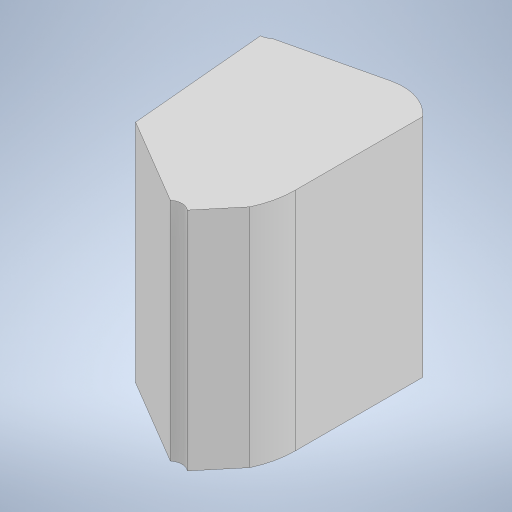
# Autodesk Inventor part: Part1
Saved by Autodesk Inventor 2024.1 (Build 281209000, 209)
## iProperties
Created: 2024-01-20
Part Number: Part1
Material: Generic
Document SubType Name: Modeling
Designer: vg3
Density: 1 g/cm^3
Appearance: Default
Author: vg3
Autodesk Inventor part; units mm, degrees
ref_plane "YZ Plane" through (0, 0, 0) normal (1, 0, 0) x (0, 1, 0)
ref_plane "XZ Plane" through (0, 0, 0) normal (0, 1, 0) x (-1, 0, 0)
ref_plane "XY Plane" through (0, 0, 0) normal (0, 0, 1) x (1, 0, 0)
sketch "Sketch1" plane through (0, 0, 0) normal (0, 1, 0) x (-1, 0, 0)
  line L0 (7.2314, 12.2227) -> (8.6145, -3.2023)
  arc A0 (8.6145, -3.2023) -> (7.6223, -3.6232) centre (8.7714, -4.952) ccw
  line L1 (7.6223, -3.6232) -> (-3.1421, -6.1489)
  arc A1 (-8.374, -4.4651) -> (-3.1421, -6.1489) centre (-4.3594, -0.9611) ccw
  line L2 (-8.374, -4.4651) -> (-8.374, 9.8774)
  arc A2 (-7.4419, 14.0569) -> (-8.374, 9.8774) centre (1.4622, 9.8774) ccw
  line L3 (-7.4419, 14.0569) -> (-4.2604, 17.8775)
  arc A3 (-4.2604, 17.8775) -> (-2.3303, 17.8775) centre (-3.2954, 19.0365) ccw
  line L4 (-2.3303, 17.8775) -> (7.2314, 12.2227)
  point P0 (0, 0)
  constraints: 10 end point, 9 point on circle, 4 centre point, 2 point on line, 2 tangent, 1 vertical
extrude "Extrusion1" add sketch "Sketch1" along normal blind 25.4
body "Solid1"
